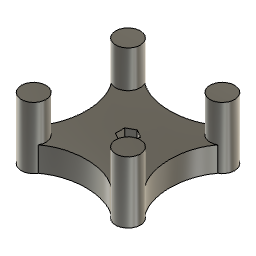
spinner (Autodesk Fusion 360 design; units mm, degrees)
Autodesk Fusion 360 part; units mm, degrees
note: some values were not read from the file. Set by a fixed rule: which sketch regions a step uses.
sketch "草图1" plane through (0, 0, 0) normal (0, 0, 1) x (1, 0, 0) in component "spinner with 4 wheel v3"
  circle A0 centre (-19.1272, 19.1272) radius 4.95
  circle A1 centre (19.1272, 19.1272) radius 4.95
  circle A2 centre (19.1272, -19.1272) radius 4.95
  circle A3 centre (-19.1272, -19.1272) radius 4.95
  ellipse E0 centre (32, 0) end of major axis (47, 0) minor radius 20.5 (21.6933, 14.8943) -> (21.6933, -14.8943) ccw
  ellipse E1 centre (0, 32) end of major axis (0, 47) minor radius 20.5 (-14.8943, 21.6933) -> (14.8943, 21.6933) ccw
  line L0 (0, 41) -> (0, 70)
  line L1 (0, -47) -> (0, -70)
  ellipse E2 centre (-32, 0) end of major axis (-17, 0) minor radius 20.5 (-21.6933, -14.8943) -> (-21.6933, 14.8943) ccw
  ellipse E3 centre (0, -32) end of major axis (0, -17) minor radius 20.5 (14.8943, -21.6933) -> (-14.8943, -21.6933) ccw
  line L2 (3.25, 1.8764) -> (0, 3.7528)
  line L3 (0, 3.7528) -> (-3.25, 1.8764)
  line L4 (-3.25, 1.8764) -> (-3.25, -1.8764)
  line L5 (-3.25, -1.8764) -> (0, -3.7528)
  line L6 (0, -3.7528) -> (3.25, -1.8764)
  line L7 (3.25, -1.8764) -> (3.25, 1.8764)
  line L8 (30, -20) -> (19.1272, -19.1272)
  dimension "d5" = 9.9
  dimension "d6" = 9.9
  dimension "d7" = 9.9
  dimension "d8" = 9.9
  dimension "d9" = 30
  dimension "d10" = 41
  dimension "d15" = 30
  dimension "d16" = 41
  dimension "d17" = 3.25
  constraint coincident A2.centre L8.end
  measures "d5" diameter of A0
  measures "d6" diameter of A1
  measures "d7" diameter of A2
  measures "d8" diameter of A3
  measures "d9" distance of E0
  measures "d15" distance of E1
  measures "d17" distance of origin L7
extrude "拉伸1" add sketch "草图1" along normal blind 5 in component "spinner with 4 wheel v3"
sketch "草图2" plane through (0, 0, 5) normal (0, 0, 1) x (-1, 0, 0) in component "spinner with 4 wheel v3"
  line L0 (-3.25, -1.8764) -> (-3.25, 1.8764)
  line L1 (-3.25, 1.8764) -> (0, 3.7528)
  line L2 (0, 3.7528) -> (3.25, 1.8764)
  line L3 (3.25, 1.8764) -> (3.25, -1.8764)
  line L4 (3.25, -1.8764) -> (0, -3.7528)
  line L5 (0, -3.7528) -> (-3.25, -1.8764)
  ellipse E0 centre (0, 32) end of major axis (20.5, 32) minor radius 15 (-14.8943, 21.6933) -> (14.8943, 21.6933) ccw
  arc A0 (-14.8943, 21.6933) -> (-21.6933, 14.8943) centre (-19.1272, 19.1272) ccw
  ellipse E1 centre (-32, 0) end of major axis (-32, -20.5) minor radius 15 (-21.6933, -14.8943) -> (-21.6933, 14.8943) ccw
  arc A1 (-21.6933, -14.8943) -> (-14.8943, -21.6933) centre (-19.1272, -19.1272) ccw
  ellipse E2 centre (0, -32) end of major axis (20.5, -32) minor radius 15 (14.8943, -21.6933) -> (-14.8943, -21.6933) ccw
  arc A2 (14.8943, -21.6933) -> (21.6933, -14.8943) centre (19.1272, -19.1272) ccw
  ellipse E3 centre (32, 0) end of major axis (32, -20.5) minor radius 15 (21.6933, 14.8943) -> (21.6933, -14.8943) ccw
  arc A3 (21.6933, 14.8943) -> (14.8943, 21.6933) centre (19.1272, 19.1272) ccw
  circle A4 centre (-19.1272, -19.1272) radius 4.95
  circle A5 centre (19.1272, -19.1272) radius 4.95
  circle A6 centre (19.1272, 19.1272) radius 4.95
  circle A7 centre (-19.1272, 19.1272) radius 4.95
  dimension "d20" = 9.9
  dimension "d21" = 4.95
  dimension "d22" = 9.9
  dimension "d23" = 4.95
  constraint concentric A1 A4
  constraint concentric A2 A5
  constraint concentric A3 A6
  constraint concentric A0 A7
  measures "d20" diameter of A1
  measures "d21" radius of A0
  measures "d22" diameter of A3
  measures "d23" radius of A2
extrude "拉伸2" add sketch "草图2" along normal blind 7 contours A0 A7 | A3 A6 | A1 A4 | A2 A5 in component "spinner with 4 wheel v3"
sketch "草图3" plane through (0, 0, 5) normal (0, 0, 1) x (-1, 0, 0) in component "spinner with 4 wheel v3"
  arc A0 (-14.8943, -21.6933) -> (-21.6933, -14.8943) centre (-19.1272, -19.1272) ccw
  ellipse E0 centre (0, -32) end of major axis (20.5, -32) minor radius 15 (14.8943, -21.6933) -> (-14.8943, -21.6933) ccw
  arc A1 (21.6933, -14.8943) -> (14.8943, -21.6933) centre (19.1272, -19.1272) ccw
  ellipse E1 centre (32, 0) end of major axis (32, -20.5) minor radius 15 (21.6933, 14.8943) -> (21.6933, -14.8943) ccw
  arc A2 (14.8943, 21.6933) -> (21.6933, 14.8943) centre (19.1272, 19.1272) ccw
  ellipse E2 centre (0, 32) end of major axis (20.5, 32) minor radius 15 (-14.8943, 21.6933) -> (14.8943, 21.6933) ccw
  arc A3 (-21.6933, 14.8943) -> (-14.8943, 21.6933) centre (-19.1272, 19.1272) ccw
  ellipse E3 centre (-32, 0) end of major axis (-32, -20.5) minor radius 15 (-21.6933, -14.8943) -> (-21.6933, 14.8943) ccw
  line L0 (-3.25, -1.8764) -> (-3.25, 1.8764)
  line L1 (-3.25, 1.8764) -> (0, 3.7528)
  line L2 (0, 3.7528) -> (3.25, 1.8764)
  line L3 (3.25, 1.8764) -> (3.25, -1.8764)
  line L4 (3.25, -1.8764) -> (0, -3.7528)
  line L5 (0, -3.7528) -> (-3.25, -1.8764)
  line L6 (-3.25, -1.8764) -> (0, -3.7528)
  line L7 (0, -3.7528) -> (3.25, -1.8764)
  line L8 (3.25, -1.8764) -> (3.25, 1.8764)
  line L9 (3.25, 1.8764) -> (0, 3.7528)
  line L10 (0, 3.7528) -> (-3.25, 1.8764)
  line L11 (-3.25, 1.8764) -> (-3.25, -1.8764)
extrude "拉伸3" add sketch "草图3" against normal blind 2 contours L0 L1 L2 L3 L4 L5 L6 L7 L8 L9 L10 L11 in component "spinner with 4 wheel v3"
sketch "草图4" plane through (0, 0, 5) normal (0, 0, 1) x (-1, 0, 0) in component "spinner with 4 wheel v3"
  arc A0 (-14.8943, -21.6933) -> (-21.6933, -14.8943) centre (-19.1272, -19.1272) ccw
  ellipse E0 centre (0, -32) end of major axis (20.5, -32) minor radius 15 (14.8943, -21.6933) -> (-14.8943, -21.6933) ccw
  arc A1 (21.6933, -14.8943) -> (14.8943, -21.6933) centre (19.1272, -19.1272) ccw
  ellipse E1 centre (32, 0) end of major axis (32, -20.5) minor radius 15 (21.6933, 14.8943) -> (21.6933, -14.8943) ccw
  arc A2 (14.8943, 21.6933) -> (21.6933, 14.8943) centre (19.1272, 19.1272) ccw
  ellipse E2 centre (0, 32) end of major axis (20.5, 32) minor radius 15 (-14.8943, 21.6933) -> (14.8943, 21.6933) ccw
  arc A3 (-21.6933, 14.8943) -> (-14.8943, 21.6933) centre (-19.1272, 19.1272) ccw
  ellipse E3 centre (-32, 0) end of major axis (-32, -20.5) minor radius 15 (-21.6933, -14.8943) -> (-21.6933, 14.8943) ccw
  circle A4 centre (0, 0) radius 2
  constraint coincident A4.centre origin
extrude "拉伸4" add sketch "草图4" along normal blind 15 contours A4 in component "spinner with 4 wheel v3"
sketch "草图5" plane through (0, 0, 0) normal (0, 0, 1) x (1, 0, 0) in component "spinner with 4 wheel v3"
extrude "拉伸5" add 1 faces at (1.0833, -0.6255, 3) along direction (0, 0, -1) blind 3 in component "spinner with 4 wheel v3"
sketch "草图6" plane through (0, 0, 0) normal (0, 0, 1) x (1, 0, 0) in component "spinner with 4 wheel v3"
  line L0 (-3.2, -1.8475) -> (0, -3.695)
  line L1 (0, -3.695) -> (3.2, -1.8475)
  line L2 (3.2, -1.8475) -> (3.2, 1.8475)
  line L3 (3.2, 1.8475) -> (0, 3.695)
  line L4 (0, 3.695) -> (-3.2, 1.8475)
  line L5 (-3.2, 1.8475) -> (-3.2, -1.8475)
  dimension "d32" = 3.2
  measures "d32" distance of origin L5
extrude "拉伸6" cut sketch "草图6" along normal blind 22 in component "spinner with 4 wheel v3"
sketch "草图7" plane through (0, 0, 0) normal (1, 0, 0) x (0, 1, 0) in component "spinner with 4 wheel v3"
extrude "拉伸7" cut 4 faces at (18.1573, 20.0862, 12) (16.979, -18.0927, 12) (-17.5166, -19.4446, 12) (-20.5586, 20.6052, 12) along direction (0, 0, -1) blind 12 in component "spinner with 4 wheel v3"
sketch "草图8" plane through (0, 0, 5) normal (0, 0, 1) x (-1, 0, 0) in component "spinner with 4 wheel v3"
  arc A0 (-14.8943, -21.6933) -> (-21.6933, -14.8943) centre (-19.1272, -19.1272) ccw
  ellipse E0 centre (0, -32) end of major axis (20.5, -32) minor radius 15 (14.8943, -21.6933) -> (-14.8943, -21.6933) ccw
  arc A1 (21.6933, -14.8943) -> (14.8943, -21.6933) centre (19.1272, -19.1272) ccw
  ellipse E1 centre (32, 0) end of major axis (32, -20.5) minor radius 15 (21.6933, 14.8943) -> (21.6933, -14.8943) ccw
  arc A2 (14.8943, 21.6933) -> (21.6933, 14.8943) centre (19.1272, 19.1272) ccw
  ellipse E2 centre (0, 32) end of major axis (20.5, 32) minor radius 15 (-14.8943, 21.6933) -> (14.8943, 21.6933) ccw
  arc A3 (-21.6933, 14.8943) -> (-14.8943, 21.6933) centre (-19.1272, 19.1272) ccw
  ellipse E3 centre (-32, 0) end of major axis (-32, -20.5) minor radius 15 (-21.6933, -14.8943) -> (-21.6933, 14.8943) ccw
  circle A4 centre (-19.1272, 19.1272) radius 5
  circle A5 centre (-19.1272, -19.1272) radius 5
  circle A6 centre (19.1272, 19.1272) radius 5
  circle A7 centre (19.1272, -19.1272) radius 5
  line L0 (3.2, -1.8475) -> (0, -3.695)
  line L1 (0, -3.695) -> (-3.2, -1.8475)
  line L2 (-3.2, -1.8475) -> (-3.2, 1.8475)
  line L3 (-3.2, 1.8475) -> (0, 3.695)
  line L4 (0, 3.695) -> (3.2, 1.8475)
  line L5 (3.2, 1.8475) -> (3.2, -1.8475)
  dimension "d37" = 4.95
  dimension "d38" = 4.95
  dimension "d39" = 4.95
  dimension "d40" = 4.95
  dimension "d41" = 10
  dimension "d42" = 10
  dimension "d43" = 10
  dimension "d44" = 10
  constraint concentric A3 A4
  constraint concentric A0 A5
  constraint concentric A2 A6
  constraint concentric A1 A7
  measures "d37" radius of A3
  measures "d38" radius of A0
  measures "d39" radius of A1
  measures "d40" radius of A2
  measures "d41" diameter of A4
  measures "d42" diameter of A5
  measures "d43" diameter of A6
  measures "d44" diameter of A7
extrude "拉伸8" add sketch "草图8" along normal blind -5 and the other way blind -7 contours A0 E0 E3 A5 | A0 E0 E3 A5 | E0 A1 E1 A7 | E0 A1 E1 A7 | E2 A3 E3 A4 | E2 A3 E3 A4 | E1 A2 E2 A6 | E1 A2 E2 A6 in component "spinner with 4 wheel v3"
extrude "拉伸9" add 4 faces at (20.5783, 17.6971, 12) (-17.6037, 17.7136, 12) (-20.6618, -20.4674, 12) (18.5183, -20.4625, 12) along direction (0, 0, 1) blind 8 in component "spinner with 4 wheel v3"
extrude "拉伸10" add 1 faces at (9.8129, -9.3621, 0) along direction (0, 0, -1) blind 5 in component "spinner with 4 wheel v3"
sketch "草图1 (2)" plane through (0, 0, 0) normal (1, 0, 0) x (0, 1, 0)
component "spinner with 4 wheel v3" placed x (1, 0, 0) y (0, 1, 0) z (0, 0, 1) at (0, 0, 0)
